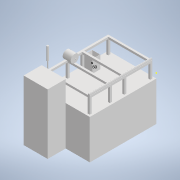
# Autodesk Inventor part: Gantry
Saved by Autodesk Inventor 2020 (Build 240168000, 168)
## iProperties
Created: 2019-10-05
Part Number: Gantry
Material: Genérico
Document SubType Name: Modeling
Designer: dasa1
Density: 1 g/cm^3
Appearance: Valor por defecto
Author: dasa1
Autodesk Inventor part; units mm, degrees
ref_plane "YZ Plane" through (0, 0, 0) normal (1, 0, 0) x (0, 1, 0)
ref_plane "XZ Plane" through (0, 0, 0) normal (0, 1, 0) x (-1, 0, 0)
ref_plane "XY Plane" through (0, 0, 0) normal (0, 0, 1) x (1, 0, 0)
sketch "Boceto1" plane through (0, 0, 0) normal (0, 1, 0) x (-1, 0, 0)
  line L0 (0, 0) -> (1200, 0)
  line L1 (1200, 0) -> (1200, 1660)
  line L2 (1200, 1660) -> (0, 1660)
  line L3 (0, 1660) -> (0, 0)
  dimension "d0" = 1200
  dimension "d1" = 1660
  constraints: 8 end point, 2 parallel, 1 horizontal, 1 perpendicular
  measures "d0" distance of L2.end L1.end
  measures "d1" distance of L1.end L0.end
extrude "Extrusión1" add sketch "Boceto1" along normal blind 1380
sketch "Boceto3" plane through (0, 1380, 0) normal (0, 1, 0) x (1, 0, 0)
  line L0 (-1200, 0) -> (-1200, -1660) projected
  line L1 (-1200, -1660) -> (0, -1660) projected
  line L2 (0, -1660) -> (0, 0) projected
  line L3 (0, 0) -> (-1200, 0) projected
  line L4 (0, -1660) -> (0, 0) construction
  line L5 (0, 0) -> (-50, 0) construction
  line L6 (-50, 0) -> (-50, -50) construction
  line L7 (-50, -50) -> (0, -50) construction
  line L8 (0, -50) -> (0, 0) construction
  line L9 (-1200, 0) -> (-1200, -1660) construction
  line L10 (-1200, -1660) -> (-1150, -1660) construction
  line L11 (-1150, -1660) -> (-1150, -1610) construction
  line L12 (-1150, -1610) -> (-1200, -1610) construction
  line L13 (-1200, -1610) -> (-1200, -1660) construction
  line L14 (-1150, -1610) -> (-1150, -50)
  line L15 (-50, -50) -> (-1150, -50)
  line L16 (-50, -50) -> (-50, -1610)
  line L17 (-50, -1610) -> (-1150, -1610)
  line L18 (-1150, -1610) -> (-50, -1610) construction
  line L19 (-50, -1610) -> (-50, -1110) construction
  line L20 (-50, -1110) -> (-1150, -1110) construction
  line L21 (-1150, -1110) -> (-1150, -1610) construction
  line L22 (-1150, -50) -> (-50, -50) construction
  line L23 (-50, -50) -> (-50, -700) construction
  line L24 (-50, -700) -> (-1150, -700) construction
  line L25 (-1150, -700) -> (-1150, -50) construction
  line L26 (-1150, -1110) -> (-1100, -1110) construction
  line L27 (-1100, -1110) -> (-1100, -1060) construction
  line L28 (-1100, -1060) -> (-1150, -1060) construction
  line L29 (-1150, -1060) -> (-1150, -1110) construction
  line L30 (-50, -700) -> (-100, -700) construction
  line L31 (-100, -700) -> (-100, -750) construction
  line L32 (-100, -750) -> (-50, -750) construction
  line L33 (-50, -750) -> (-50, -700) construction
  line L34 (-1150, -50) -> (-1100, -50) construction
  line L35 (-1100, -50) -> (-1100, -100) construction
  line L36 (-1100, -100) -> (-1150, -100) construction
  line L37 (-1150, -100) -> (-1150, -50) construction
  line L38 (-50, -1610) -> (-100, -1610) construction
  line L39 (-100, -1610) -> (-100, -1560) construction
  line L40 (-100, -1560) -> (-50, -1560) construction
  line L41 (-50, -1560) -> (-50, -1610) construction
  line L42 (-100, -1560) -> (-1100, -1560)
  line L43 (-1100, -1560) -> (-1100, -1110)
  line L44 (-1100, -1110) -> (-100, -1110)
  line L45 (-100, -1110) -> (-100, -1560)
  line L46 (-1100, -1060) -> (-100, -1060)
  line L47 (-100, -1060) -> (-100, -750)
  line L48 (-100, -750) -> (-1100, -750)
  line L49 (-1100, -750) -> (-1100, -1060)
  line L50 (-100, -700) -> (-1100, -700)
  line L51 (-1100, -700) -> (-1100, -100)
  line L52 (-1100, -100) -> (-100, -100)
  line L53 (-100, -100) -> (-100, -700)
  dimension "d7" = 50
  dimension "d8" = 50
  dimension "d9" = 50
  dimension "d10" = 50
  dimension "d13" = 500
  dimension "d14" = 650
  dimension "d15" = 50
  dimension "d16" = 50
  dimension "d17" = 50
  dimension "d18" = 50
  dimension "d19" = 50
  dimension "d20" = 50
  dimension "d21" = 50
  dimension "d22" = 50
  constraints: 96 end point, 23 parallel, 13 perpendicular, 11 horizontal, 2 point on line, 1 vertical
  measures "d7" distance of L7.end L6.end
  measures "d8" distance of L6.end L5.end
  measures "d9" distance of L12.end L11.end
  measures "d10" distance of L11.end L10.end
  measures "d13" distance of L19.end L18.end
  measures "d14" distance of L22.end L23.end
  measures "d15" distance of L28.end L27.end
  measures "d16" distance of L27.end L26.end
  measures "d17" distance of L32.end L31.end
  measures "d18" distance of L31.end L30.end
  measures "d19" distance of L35.end L36.end
  measures "d20" distance of L34.end L35.end
  measures "d21" distance of L39.end L40.end
  measures "d22" distance of L38.end L39.end
extrude "Extrusión2" cut sketch "Boceto3" against normal blind 400
sketch "Boceto4" plane through (-50, 1380, 1610) normal (1, 0, 0) x (0, 0, -1)
  line L0 (50, 0) -> (500, 0) construction
  line L1 (50, 0) -> (50, -400) construction
  line L2 (50, -400) -> (500, -400) construction
  line L3 (500, 0) -> (500, -400) construction
  line L4 (550, 0) -> (860, 0) construction
  line L5 (550, 0) -> (550, -400) construction
  line L6 (550, -400) -> (860, -400) construction
  line L7 (860, 0) -> (860, -400) construction
  line L8 (910, 0) -> (1510, 0) construction
  line L9 (910, 0) -> (910, -400) construction
  line L10 (910, -400) -> (1510, -400) construction
  line L11 (1510, 0) -> (1510, -400) construction
  line L12 (50, 0) -> (500, 0) construction
  line L13 (500, 0) -> (500, -50) construction
  line L14 (500, -50) -> (50, -50) construction
  line L15 (50, -50) -> (50, 0) construction
  line L16 (550, 0) -> (860, 0) construction
  line L17 (860, 0) -> (860, -400) construction
  line L18 (550, 0) -> (860, 0) construction
  line L19 (860, 0) -> (860, -50) construction
  line L20 (860, -50) -> (550, -50) construction
  line L21 (550, -50) -> (550, 0) construction
  line L22 (910, 0) -> (910, -400) construction
  line L23 (910, 0) -> (1510, 0) construction
  line L24 (1510, 0) -> (1510, -50) construction
  line L25 (1510, -50) -> (910, -50) construction
  line L26 (910, -50) -> (910, 0) construction
  line L27 (50, -50) -> (500, -50)
  line L28 (500, -50) -> (500, -400)
  line L29 (500, -400) -> (50, -400)
  line L30 (50, -400) -> (50, -50)
  line L31 (550, -50) -> (860, -50)
  line L32 (860, -50) -> (860, -400)
  line L33 (860, -400) -> (550, -400)
  line L34 (550, -400) -> (550, -50)
  line L35 (910, -50) -> (1510, -50)
  line L36 (1510, -50) -> (1510, -400)
  line L37 (1510, -400) -> (910, -400)
  line L38 (910, -400) -> (910, -50)
  point P0 (1610, -1380)
  dimension "d23" = 50
  dimension "d24" = 50
  dimension "d25" = 50
  constraints: 48 end point, 12 parallel, 6 horizontal, 6 perpendicular, 3 point on line
  measures "d23" distance of L12.end L13.end
  measures "d24" distance of L18.end L19.end
  measures "d25" distance of L23.end L24.end
extrude "Extrusión3" cut sketch "Boceto4" against normal blind 1100
sketch "Boceto5" plane through (-1150, 1380, 1610) normal (0, 0, 1) x (1, 0, 0)
  line L0 (0, 0) -> (1100, 0) construction
  line L1 (0, 0) -> (0, -400) construction
  line L2 (0, -400) -> (1100, -400) construction
  line L3 (1100, 0) -> (1100, -400) construction
  line L4 (0, 0) -> (1100, 0) construction
  line L5 (0, 0) -> (50, 0) construction
  line L6 (50, -50) -> (0, -50) construction
  line L7 (0, -50) -> (0, 0) construction
  line L8 (1100, 0) -> (1050, 0) construction
  line L9 (1050, 0) -> (1050, -50) construction
  line L10 (1050, -50) -> (1100, -50) construction
  line L11 (1100, -50) -> (1100, 0) construction
  line L12 (1100, -400) -> (0, -400) projected
  line L13 (50, -50) -> (1050, -50)
  line L14 (1050, -50) -> (1050, -400)
  line L15 (1050, -400) -> (50, -400)
  line L16 (50, -400) -> (50, -50)
  point P0 (1150, -1380)
  dimension "d29" = 50
  dimension "d30" = 50
  dimension "d31" = 50
  dimension "d32" = 50
  constraints: 22 end point, 5 parallel, 3 horizontal, 2 perpendicular, 1 point on line
  measures "d29" distance of L5.end L6.start
  measures "d30" distance of L10.end L9.end
  measures "d31" distance of L9.end L8.end
  measures "d32" distance from line of L13.end L3
extrude "Extrusión4" cut sketch "Boceto5" against normal blind 1600
sketch "Boceto6" plane through (0, 1380, 0) normal (0, 1, 0) x (1, 0, 0)
  line L0 (-1100, -700) -> (-1100, -100) construction
  line L1 (-1100, -100) -> (-100, -100) construction
  line L2 (-100, -100) -> (-100, -700) construction
  line L3 (-100, -700) -> (-1100, -700) construction
  line L4 (-100, -1060) -> (-1100, -1060) construction
  line L5 (-1100, -1060) -> (-1100, -750) construction
  line L6 (-1100, -750) -> (-100, -750) construction
  line L7 (-100, -750) -> (-100, -1060) construction
  line L8 (-50, -1610) -> (-50, -50) construction
  line L9 (-50, -50) -> (-1150, -50) construction
  line L10 (-1150, -50) -> (-1150, -1610) construction
  line L11 (-1150, -1610) -> (-50, -1610) construction
  line L12 (-1100, -1560) -> (-1100, -1110) construction
  line L13 (-1100, -1110) -> (-100, -1110) construction
  line L14 (-100, -1110) -> (-100, -1560) construction
  line L15 (-100, -1560) -> (-1100, -1560) construction
  line L16 (-50, -1060) -> (-100, -1060) construction
  line L17 (-50, -1110) -> (-50, -1060) construction
  line L18 (-50, -1110) -> (-100, -1110) construction
  line L19 (-100, -1110) -> (-100, -1060) construction
  line L20 (-1100, -750) -> (-1150, -750) construction
  line L21 (-1150, -700) -> (-1150, -750) construction
  line L22 (-1100, -700) -> (-1150, -700) construction
  line L23 (-1100, -750) -> (-1100, -700) construction
  line L24 (-50, -1560) -> (-100, -1560) construction
  line L25 (-50, -1610) -> (-50, -1560) construction
  line L26 (-100, -1610) -> (-50, -1610) construction
  line L27 (-100, -1610) -> (-100, -1560) construction
  line L28 (-1100, -100) -> (-1150, -100) construction
  line L29 (-1150, -50) -> (-1150, -100) construction
  line L30 (-1100, -50) -> (-1150, -50) construction
  line L31 (-1100, -100) -> (-1100, -50) construction
  line L32 (-100, -750) -> (-100, -700) construction
  line L33 (-50, -700) -> (-100, -700) construction
  line L34 (-50, -750) -> (-50, -700) construction
  line L35 (-50, -750) -> (-100, -750) construction
  line L36 (-1100, -1110) -> (-1100, -1060) construction
  line L37 (-1100, -1110) -> (-1150, -1110) construction
  line L38 (-1150, -1060) -> (-1150, -1110) construction
  line L39 (-1100, -1060) -> (-1150, -1060) construction
  line L40 (-1100, -1610) -> (-1100, -1560) construction
  line L41 (-1150, -1610) -> (-1100, -1610) construction
  line L42 (-1150, -1560) -> (-1150, -1610) construction
  line L43 (-1100, -1560) -> (-1150, -1560) construction
  line L44 (0, -1660) -> (-1200, -1660) construction
  line L45 (0, 0) -> (0, -1660) construction
  line L46 (-1200, 0) -> (0, 0) construction
  line L47 (-1200, -1660) -> (-1200, 0) construction
  line L48 (-100, -100) -> (-100, -50) construction
  line L49 (-50, -50) -> (-100, -50) construction
  line L50 (-50, -100) -> (-50, -50) construction
  line L51 (-50, -100) -> (-100, -100) construction
  line L52 (-50, -50) -> (-1150, -50) construction
  line L53 (-100, -1610) -> (-95, -1610) construction
  line L54 (-95, -1610) -> (-95, -50) construction
  line L55 (-95, -50) -> (-100, -50) construction
  line L56 (-100, -50) -> (-100, -1610) construction
  line L57 (-1150, -1610) -> (-50, -1610) construction
  line L58 (-50, -50) -> (-55, -50) construction
  line L59 (-55, -50) -> (-55, -1610) construction
  line L60 (-55, -1610) -> (-50, -1610) construction
  line L61 (-50, -1610) -> (-50, -50) construction
  line L62 (-55, -1610) -> (-95, -1610)
  line L63 (-95, -1610) -> (-95, -50)
  line L64 (-95, -50) -> (-55, -50)
  line L65 (-55, -50) -> (-55, -1610)
  dimension "d35" = 5
  dimension "d36" = 5
  constraints: 24 end point, 6 parallel, 3 horizontal, 3 perpendicular, 2 point on line
  measures "d35" distance of L55.end L54.end
  measures "d36" distance of L60.end L59.end
extrude "Extrusión5" add sketch "Boceto6" along normal blind 40
sketch "Boceto7" plane through (-1150, 1380, 50) normal (-1, 0, 0) x (0, 0, 1)
  line L0 (650, -50) -> (650, -400) construction
  line L1 (650, -400) -> (700, -400) construction
  line L2 (700, -400) -> (700, -50) construction
  line L3 (700, -50) -> (1010, -50) construction
  line L4 (1010, -50) -> (1010, -400) construction
  line L5 (1010, -400) -> (1060, -400) construction
  line L6 (1060, -400) -> (1060, -50) construction
  line L7 (1060, -50) -> (1510, -50) construction
  line L8 (1510, -50) -> (1510, -400) construction
  line L9 (1510, -400) -> (1560, -400) construction
  line L10 (1560, 0) -> (1560, -400) construction
  line L11 (0, 0) -> (1560, 0) construction
  line L12 (0, 0) -> (0, -400) construction
  line L13 (0, -400) -> (50, -400) construction
  line L14 (50, -400) -> (50, -50) construction
  line L15 (50, -50) -> (650, -50) construction
  line L16 (1010, -50) -> (700, -50) construction
  line L17 (1010, -50) -> (1035, -50) construction
  line L18 (1060, -50) -> (1010, -50) construction
  line L19 (1035, -50) -> (1035, 100) construction
  circle A0 centre (1035, 100) radius 100
  point P0 (-50, -1380)
  dimension "d40" = 150
  dimension "d41" = 200
  constraints: 4 end point, 1 centre point, 1 coincident, 1 midpoint, 1 perpendicular
  measures "d40" distance of L17.end L19.end
  measures "d41" diameter of A0
extrude "Extrusión6" add sketch "Boceto7" against normal blind 200
sketch "Boceto9" plane through (-950, 1480, 1085) normal (1, 0, 0) x (0, 0, -1)
  circle A0 centre (0, 0) radius 100 construction
  circle A1 centre (0, 0) radius 7.5
  point P0 (1085, -1480)
  point P1 (0, -100)
  dimension "d44" = 15
  constraints: 1 centre point, 1 coincident, 1 vertical alignment
  measures "d44" diameter of A1
extrude "Extrusión7" add sketch "Boceto9" along normal blind 50
fillet "Empalme1" radius 20 2 edges at (-55, 1420, 830) (-95, 1420, 830)
sketch "Boceto10" plane through (0, 1380, 0) normal (0, 1, 0) x (1, 0, 0)
  line L0 (-1100, -1610) -> (-1100, -1560) construction
  line L1 (-1100, -1560) -> (-1125, -1560) construction
  line L2 (-1125, -1560) -> (-1125, -1585) construction
  line L3 (-1125, -1585) -> (-1100, -1585) construction
  line L4 (-1100, -1585) -> (-1100, -1560) construction
  circle A0 centre (-1125, -1585) radius 10
  point P0 (0, 0)
  dimension "d48" = 25
  dimension "d49" = 25
  dimension "d50" = 20
  constraints: 8 end point, 2 parallel, 1 centre point, 1 coincident, 1 horizontal, 1 perpendicular
  measures "d48" distance of L3.end L2.end
  measures "d49" distance of L2.end L1.end
  measures "d50" diameter of A0
extrude "Extrusión8" add sketch "Boceto10" along normal blind 220
sketch "Boceto11" plane through (-1125, 1600, 1585) normal (0, 1, 0) x (1, 0, 0)
  circle A0 centre (0, 0) radius 10 construction
  circle A1 centre (0, 0) radius 25
  line L0 (25, -25) -> (25, 25) projected
  point P0 (1125, 1585)
  constraints: 1 centre point, 1 coincident, 1 tangent
extrude "Extrusión9" add sketch "Boceto11" along normal blind 320
sketch "Boceto12" plane through (0, 980, 0) normal (0, 1, 0) x (1, 0, 0)
  line L0 (-1100, -750) -> (-1100, -700) projected
  line L1 (-1100, -700) -> (-900, -700)
  line L2 (-900, -700) -> (-900, -500)
  line L3 (-900, -500) -> (-1100, -500)
  line L4 (-1100, -500) -> (-1100, -700)
  point P0 (0, 0)
  dimension "d55" = 200
  dimension "d56" = 200
  constraints: 8 end point, 2 parallel, 1 horizontal, 1 perpendicular
  measures "d55" distance of L3.end L2.end
  measures "d56" distance of L2.end L1.end
extrude "Extrusión10" add sketch "Boceto12" along normal blind 120
sketch "Boceto13" plane through (0, 1100, 0) normal (0, 1, 0) x (1, 0, 0)
  line L0 (-100, -700) -> (-1100, -700) projected
  line L1 (-900, -500) -> (-1100, -500) projected
  line L2 (-1100, -700) -> (-900, -700)
  line L3 (-900, -700) -> (-900, -500)
  line L4 (-900, -500) -> (-1100, -500)
  line L5 (-1100, -500) -> (-1100, -700)
  point P0 (0, 0)
  constraints: 8 end point, 2 parallel, 1 horizontal, 1 perpendicular
extrude "Extrusión11" add sketch "Boceto13" along normal blind 200
sketch "Boceto14" plane through (0, 1300, 0) normal (0, 1, 0) x (1, 0, 0)
  line L0 (-1100, -500) -> (-1100, -700) construction
  line L1 (-1100, -700) -> (-900, -700) construction
  line L2 (-900, -700) -> (-900, -500) construction
  line L3 (-900, -500) -> (-1100, -500) construction
  line L4 (-1100, -750) -> (-1100, -700) construction
  line L5 (-1100, -700) -> (-1050, -700) construction
  line L6 (-1050, -700) -> (-1050, -650) construction
  line L7 (-1050, -650) -> (-1100, -650) construction
  line L8 (-1100, -650) -> (-1100, -700) construction
  line L9 (-900, -500) -> (-900, -700) construction
  line L10 (-900, -500) -> (-950, -500) construction
  line L11 (-950, -500) -> (-950, -550) construction
  line L12 (-950, -550) -> (-900, -550) construction
  line L13 (-900, -550) -> (-900, -500) construction
  line L14 (-1050, -650) -> (-950, -650)
  line L15 (-950, -650) -> (-950, -550)
  line L16 (-950, -550) -> (-1050, -550)
  line L17 (-1050, -550) -> (-1050, -650)
  point P0 (0, 0)
  dimension "d61" = 50
  dimension "d62" = 50
  dimension "d63" = 50
  dimension "d64" = 50
  dimension "d65" = 100
  dimension "d66" = 100
  constraints: 24 end point, 6 parallel, 3 horizontal, 3 perpendicular
  measures "d61" distance of L7.end L6.end
  measures "d62" distance of L6.end L5.end
  measures "d63" distance of L12.end L11.end
  measures "d64" distance of L11.end L10.end
  measures "d65" distance of L16.end L11.end
  measures "d66" distance of L11.end L14.end
extrude "Extrusión12" cut sketch "Boceto14" against normal blind 200
draft "Cara para el ángulo de desmoldeo1" angle 13 pull direction (0, 1, 0) faces at (-1016.6667, 1233.3333, 650) fixed edges at (-1000, 1100, 650)
draft "Cara para el ángulo de desmoldeo2" angle 13 pull direction (0, 1, 0) fixed plane through (-1016.6667, 1100, 583.3333) normal (0, 1, 0) faces at (-1050, 1233.3333, 632.0579)
draft "Cara para el ángulo de desmoldeo3" angle 13 pull direction (0, 1, 0) fixed plane through (-1016.6667, 1100, 583.3333) normal (0, 1, 0) faces at (-950, 1233.3333, 632.0579)
draft "Cara para el ángulo de desmoldeo4" angle 13 pull direction (0, 1, 0) fixed plane through (-1016.6667, 1100, 583.3333) normal (0, 1, 0) faces at (-983.3333, 1233.3333, 550)
sketch "Boceto15" plane through (0, 0, 0) normal (0, -1, 0) x (1, 0, 0)
  line L0 (-1200, 0) -> (-1200, 1660) construction
  line L1 (0, 0) -> (-1200, 0) construction
  line L2 (0, 1660) -> (0, 0) construction
  line L3 (-1200, 1660) -> (0, 1660) construction
  line L4 (-1200, 1660) -> (0, 1660) projected
  line L5 (-1200, 1660) -> (-600, 1660)
  line L6 (-600, 1660) -> (-600, 2110)
  line L7 (-600, 2110) -> (-1200, 2110)
  line L8 (-1200, 2110) -> (-1200, 1660)
  dimension "d73" = 600
  dimension "d74" = 450
  constraints: 8 end point, 2 parallel, 1 horizontal, 1 perpendicular
  measures "d73" distance of L7.end L6.end
  measures "d74" distance of L6.end L5.end
extrude "Extrusión13" add sketch "Boceto15" against normal blind 1500
sketch "Boceto16" plane through (0, 1100, 0) normal (0, 1, 0) x (1, 0, 0)
  line L0 (-950, -650) -> (-1050, -650) projected
  line L1 (-950, -550) -> (-950, -650) projected
  line L2 (-1050, -550) -> (-950, -550) projected
  line L3 (-1050, -650) -> (-1050, -550) projected
  circle A0 centre (-1000, -600) radius 30
  point P0 (0, 0)
  dimension "d77" = 60
  constraints: 1 centre point
  measures "d77" diameter of A0
